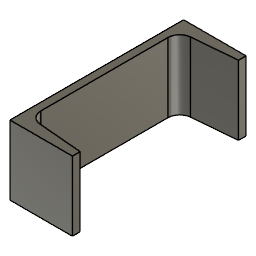
C-250×90×11×14.5 (Autodesk Fusion 360 design; units mm, degrees)
Autodesk Fusion 360 part; units mm, degrees
note: some values were not read from the file. Set by a fixed rule: which sketch regions a step uses.
sketch "スケッチ1" plane through (0, 0, 0) normal (0, 0, 1) x (1, 0, 0)
  line L0 (0, 250) -> (0, 0)
  line L1 (0, 0) -> (90, 0)
  line L2 (90, 11.0442) -> (90, 0)
  line L3 (26.5184, 16.5981) -> (90, 11.0442)
  line L4 (90, 238.9558) -> (26.5184, 233.4019)
  line L5 (0, 250) -> (90, 250)
  line L6 (11, 216.4666) -> (11, 33.5334)
  arc A0 (11, 33.5334) -> (26.5184, 16.5981) centre (28, 33.5334) ccw
  arc A1 (26.5184, 233.4019) -> (11, 216.4666) centre (28, 216.4666) ccw
  line L7 (90, 250) -> (90, 238.9558)
extrude "押し出し1" add sketch "スケッチ1" along normal blind 100
